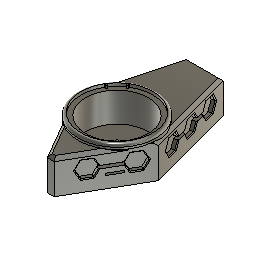
wedge_15deg_18mm_cirque (Autodesk Fusion 360 design; units mm, degrees)
Autodesk Fusion 360 part; units mm, degrees
sketch "wedge-base" plane through (0, 0, 0) normal (0, 0, 1) x (1, 0, 0)
  line L0 (-31.305, -84.6876) -> (-19.8752, -42.031)
  line L1 (-139.1957, -104.8346) -> (-25.4147, -135.3221)
  line L2 (-74.9975, -19.3163) -> (-95.8937, -18.9648)
  line L3 (-118.0318, -25.8497) -> (-139.1957, -104.8346)
  line L4 (-95.8937, -18.9648) -> (-118.0318, -25.8497)
  line L5 (-12.6022, -117.024) -> (-31.305, -84.6876)
  line L6 (-19.8752, -42.031) -> (-56.3483, -24.332)
  line L7 (-56.3483, -24.332) -> (-56.434, -24.2904)
  line L8 (-25.4147, -135.3221) -> (-12.6022, -117.024)
  line L9 (-56.434, -24.2904) -> (-74.9975, -19.3163)
  line L10 (-55.3814, -21.4666) -> (-74.5778, -16.323)
  line L11 (-24.1621, -138.7635) -> (-9.0476, -117.1778)
  line L12 (-120.5016, -23.4761) -> (-142.8699, -106.9559)
  line L13 (-16.336, -40.4139) -> (-55.3814, -21.4666)
  line L14 (-74.5778, -16.323) -> (-96.3248, -15.9571)
  line L15 (-9.0476, -117.1778) -> (-28.0852, -84.2624)
  line L16 (-28.0852, -84.2624) -> (-16.336, -40.4139)
  line L17 (-96.3248, -15.9571) -> (-120.5016, -23.4761)
  line L18 (-142.8699, -106.9559) -> (-24.1621, -138.7635)
  line L19 (-30.0171, -84.5175) -> (-18.4595, -41.3841)
  line L20 (-119.0197, -24.9003) -> (-140.6654, -105.6831)
  line L21 (-24.9136, -136.6987) -> (-11.1804, -117.0855)
  line L22 (-96.0662, -17.7617) -> (-119.0197, -24.9003)
  line L23 (-18.4595, -41.3841) -> (-56.013, -23.1609)
  line L24 (-140.6654, -105.6831) -> (-24.9136, -136.6987)
  line L25 (-56.013, -23.1609) -> (-74.8297, -18.119)
  line L26 (-11.1804, -117.0855) -> (-30.0171, -84.5175)
  line L27 (-74.8297, -18.119) -> (-96.0662, -17.7617)
  line L28 (-55.5625, -22.7126) -> (-55.8025, -22.5961)
  line L29 (-29.3731, -84.4325) -> (-17.7517, -41.0607)
  line L30 (-55.8025, -22.5961) -> (-74.7457, -17.5203)
  line L31 (-17.7517, -41.0607) -> (-55.5625, -22.7126)
  line L32 (-74.7457, -17.5203) -> (-96.1524, -17.1602)
  line L33 (-119.5136, -24.4255) -> (-141.4002, -106.1074)
  line L34 (-10.4694, -117.1163) -> (-29.3731, -84.4325)
  line L35 (-141.4002, -106.1074) -> (-24.6631, -137.387)
  line L36 (-24.6631, -137.387) -> (-10.4694, -117.1163)
  line L37 (-96.1524, -17.1602) -> (-119.5136, -24.4255)
  circle A0 centre (-97.5457, -40.1917) radius 2.2
  circle A1 centre (-107.3808, -76.8969) radius 2.2
  circle A2 centre (-47.3176, -53.6503) radius 2.2
  circle A3 centre (-43.0743, -100.1574) radius 2.2
  line L38 (-104.5834, -110.8892) -> (-99.9246, -93.5026)
  line L39 (-136.4589, -102.3482) -> (-104.5834, -110.8892)
  line L40 (-99.9246, -93.5026) -> (-131.8002, -84.9615)
  line L41 (-131.8002, -84.9615) -> (-136.4589, -102.3482)
  line L42 (-100.5004, -109.2708) -> (-102.0145, -114.9215)
  line L43 (-93.5143, -117.1991) -> (-92.0002, -111.5484)
  line L44 (-92.0002, -111.5484) -> (-100.5004, -109.2708)
  line L45 (-82.5358, -118.7276) -> (-81.63, -115.3469)
  line L46 (-90.3233, -113.0175) -> (-91.2292, -116.3983)
  line L47 (-81.63, -115.3469) -> (-90.3233, -113.0175)
  line L48 (-91.2292, -116.3983) -> (-82.5358, -118.7276)
  line L49 (-21.0709, -104.8602) -> (-26.5709, -95.3339)
  line L50 (-28.9517, -109.4102) -> (-21.0709, -104.8602)
  line L51 (-26.5709, -95.3339) -> (-34.4517, -99.8839)
  line L52 (-34.4517, -99.8839) -> (-28.9517, -109.4102)
  line L53 (-107.7035, -88.1467) -> (-99.3965, -90.3726)
  line L54 (-99.3965, -90.3726) -> (-97.093, -81.7758)
  line L55 (-97.093, -81.7758) -> (-105.4, -79.55)
  line L56 (-105.4, -79.55) -> (-107.7035, -88.1467)
  line L57 (-7.336, -20.2677) -> (-7.336, -143.1078) construction
  line L58 (3.7874, -41.3841) -> (41.3409, -23.1609)
  line L59 (126.7282, -106.1074) -> (9.991, -137.387)
  line L60 (-7.336, -20.2677) -> (-7.336, -143.1078) construction
  line L61 (10.2415, -136.6987) -> (-3.4917, -117.0855)
  line L62 (41.1304, -22.5961) -> (60.0736, -17.5203)
  line L63 (11.8988, -95.3339) -> (19.7796, -99.8839)
  line L64 (105.8295, -23.4761) -> (128.1978, -106.9559)
  line L65 (19.7796, -99.8839) -> (14.2796, -109.4102)
  line L66 (41.3409, -23.1609) -> (60.1576, -18.119)
  line L67 (15.345, -84.5175) -> (3.7874, -41.3841)
  line L68 (40.7094, -21.4666) -> (59.9057, -16.323)
  line L69 (78.8422, -117.1991) -> (77.3281, -111.5484)
  line L70 (-3.4917, -117.0855) -> (15.345, -84.5175)
  line L71 (76.5571, -116.3983) -> (67.8638, -118.7276)
  line L72 (-4.2026, -117.1163) -> (14.7011, -84.4325)
  line L73 (16.6329, -84.6876) -> (5.2031, -42.031)
  line L74 (85.2525, -93.5026) -> (117.1281, -84.9615)
  line L75 (81.3941, -17.7617) -> (104.3476, -24.9003)
  line L76 (75.6512, -113.0175) -> (76.5571, -116.3983)
  line L77 (66.9579, -115.3469) -> (75.6512, -113.0175)
  circle A4 centre (32.6455, -53.6503) radius 2.2
  line L78 (89.9113, -110.8892) -> (85.2525, -93.5026)
  line L79 (14.7011, -84.4325) -> (3.0796, -41.0607)
  line L80 (67.8638, -118.7276) -> (66.9579, -115.3469)
  line L81 (128.1978, -106.9559) -> (9.49, -138.7635)
  line L82 (81.4803, -17.1602) -> (104.8416, -24.4255)
  line L83 (13.4132, -84.2624) -> (1.664, -40.4139)
  circle A5 centre (92.7087, -76.8969) radius 2.2
  line L84 (10.7426, -135.3221) -> (-2.0699, -117.024)
  line L85 (93.0314, -88.1467) -> (84.7244, -90.3726)
  line L86 (104.3476, -24.9003) -> (125.9933, -105.6831)
  line L87 (1.664, -40.4139) -> (40.7094, -21.4666)
  line L88 (90.7279, -79.55) -> (93.0314, -88.1467)
  line L89 (81.2217, -18.9648) -> (103.3597, -25.8497)
  line L90 (3.0796, -41.0607) -> (40.8904, -22.7126)
  line L91 (125.9933, -105.6831) -> (10.2415, -136.6987)
  line L92 (-2.0699, -117.024) -> (16.6329, -84.6876)
  line L93 (84.7244, -90.3726) -> (82.421, -81.7758)
  line L94 (81.6527, -15.9571) -> (105.8295, -23.4761)
  line L95 (9.991, -137.387) -> (-4.2026, -117.1163)
  line L96 (121.7868, -102.3482) -> (89.9113, -110.8892)
  line L97 (60.0736, -17.5203) -> (81.4803, -17.1602)
  line L98 (59.9057, -16.323) -> (81.6527, -15.9571)
  line L99 (6.3988, -104.8602) -> (11.8988, -95.3339)
  line L100 (82.421, -81.7758) -> (90.7279, -79.55)
  circle A6 centre (28.4022, -100.1574) radius 2.2
  line L101 (60.1576, -18.119) -> (81.3941, -17.7617)
  line L102 (41.6762, -24.332) -> (41.7619, -24.2904)
  line L103 (9.49, -138.7635) -> (-5.6245, -117.1778)
  line L104 (41.7619, -24.2904) -> (60.3255, -19.3163)
  circle A7 centre (82.8736, -40.1917) radius 2.2
  line L105 (40.8904, -22.7126) -> (41.1304, -22.5961)
  line L106 (-5.6245, -117.1778) -> (13.4132, -84.2624)
  line L107 (124.5236, -104.8346) -> (10.7426, -135.3221)
  line L108 (117.1281, -84.9615) -> (121.7868, -102.3482)
  line L109 (14.2796, -109.4102) -> (6.3988, -104.8602)
  line L110 (104.8416, -24.4255) -> (126.7282, -106.1074)
  line L111 (103.3597, -25.8497) -> (124.5236, -104.8346)
  line L112 (5.2031, -42.031) -> (41.6762, -24.332)
  line L113 (77.3281, -111.5484) -> (85.8283, -109.2708)
  line L114 (85.8283, -109.2708) -> (87.3424, -114.9215)
  line L115 (60.3255, -19.3163) -> (81.2217, -18.9648)
  line L116 (-28.0852, -84.2624) -> (13.4132, -84.2624) construction
  line L117 (-16.336, -40.4139) -> (1.664, -40.4139)
  line L118 (-9.0476, -117.1778) -> (-5.6245, -117.1778)
  point P0 (-7.336, -84.2624)
  dimension "d1" = 9
  dimension "d2" = 9
  constraint vertical L57
  constraint horizontal L116
  constraint midpoint L116 P0
  constraint coincident L13.start L16.end
  constraint perpendicular L57 L117
  constraint parallel L117 L118
  measures "d1" distance of L13.start L57
  measures "d2" distance of L83.end L60
extrude "Extrude1" add sketch "wedge-base" along normal blind 16.6 contours L15 L16 L83 L106 L117 L118
sketch "cirque" plane through (0, 0, 0) normal (0, 0, 1) x (1, 0, 0)
  arc A0 (-17.2299, -69.4279) -> (-22.1706, -74.3686) centre (-7.336, -84.2624) ccw
  arc A1 (4.4021, -96.566) -> (4.9675, -96.0005) centre (4.6848, -96.2833) cw
  arc A2 (-21.4728, -74.8131) -> (-21.8745, -75.4436) centre (-21.6737, -75.1283) cw
  arc A3 (-16.1549, -69.7239) -> (-16.7854, -70.1256) centre (-16.4701, -69.9248) cw
  line L0 (4.9675, -96.0005) -> (5.5521, -96.5851)
  arc A4 (-22.5723, -74.9991) -> (4.9867, -97.1506) centre (-7.336, -84.2624) ccw
  line L1 (-22.1706, -74.3686) -> (-21.4728, -74.8131)
  line L2 (-16.7854, -70.1256) -> (-17.2299, -69.4279)
  line L3 (4.9867, -97.1506) -> (4.4021, -96.566)
  line L4 (-21.8745, -75.4436) -> (-22.5723, -74.9991)
  arc A5 (5.5521, -96.5851) -> (-16.5994, -69.0262) centre (-7.336, -84.2624) ccw
  line L5 (-16.5994, -69.0262) -> (-16.1549, -69.7239)
  circle A6 centre (-7.336, -84.2624) radius 15.5
  line L6 (-7.336, -66.2625) -> (-7.336, -66.5624)
  circle A7 centre (-7.336, -84.2624) radius 19.3
  point P0 (-7.336, -84.2624)
  dimension "d3" = 3.8
extrude "Extrude2" cut sketch "cirque" along normal up to surface (13.6 mm away) from surface at 3 contours A6
extrude "Extrude3" add sketch "cirque" along normal blind 1 from surface at 16.6 contours A0 A1 A2 A3 L0 A4 L1 L2 L3 L4 A5 L5
extrude "Extrude5" add sketch "cirque" along normal blind 2.5 from surface at 16.6 contours A7
sketch "Sketch6" plane through (46.5701, -26.9353, 0) normal (0.865639, -0.500669, 0) x (0.500669, 0.865639, 0)
  line L0 (-104.2497, 0) -> (-66.2253, 0)
  line L1 (-66.2253, 0) -> (-66.2253, 16.6)
  line L2 (-66.2253, 16.6) -> (-69.5511, 16.6)
  line L3 (-69.5511, 16.6) -> (-83.6764, 16.6)
  line L4 (-83.6764, 16.6) -> (-104.2497, 16.6)
  line L5 (-104.2497, 16.6) -> (-104.2497, 0)
  line L6 (-85.5673, 5.7) -> (-85.5673, 6.7)
  line L7 (-85.5673, 6.7) -> (-78.5673, 6.7)
  line L8 (-78.5673, 5.7) -> (-85.5673, 5.7)
  line L9 (-78.5673, 6.7) -> (-78.5673, 5.7)
  line L10 (-104.2497, 16.6) -> (-104.2497, 2)
  line L11 (-104.2497, 2) -> (-66.2253, 2)
  line L12 (-66.2253, 16.6) -> (-104.2497, 16.6)
  line L13 (-66.2253, 2) -> (-66.2253, 16.6)
  line L14 (-89.961, 5.7214) -> (-87.6598, 9.6927)
  line L15 (-94.5383, 13.6786) -> (-96.8396, 9.7073)
  line L16 (-87.6598, 9.6927) -> (-89.9484, 13.6713)
  line L17 (-96.8396, 9.7073) -> (-94.551, 5.7287)
  line L18 (-94.551, 5.7287) -> (-89.961, 5.7214)
  line L19 (-89.9484, 13.6713) -> (-94.5383, 13.6786)
  line L20 (-71.9366, 13.6786) -> (-76.5266, 13.6713)
  line L21 (-69.6354, 9.7073) -> (-71.9366, 13.6786)
  line L22 (-71.924, 5.7287) -> (-69.6354, 9.7073)
  line L23 (-78.8152, 9.6927) -> (-76.5139, 5.7214)
  line L24 (-76.5266, 13.6713) -> (-78.8152, 9.6927)
  line L25 (-76.5139, 5.7214) -> (-71.924, 5.7287)
  arc A0 (-92.2497, 10.45) -> (-92.2497, 8.95) centre (-92.2497, 9.7) ccw
  line L26 (-92.2497, 8.95) -> (-74.2253, 8.95)
  line L27 (-74.2253, 10.45) -> (-92.2497, 10.45)
  arc A1 (-74.2253, 8.95) -> (-74.2253, 10.45) centre (-74.2253, 9.7) ccw
  point P0 (-92.2497, 9.7)
  point P1 (-74.2253, 9.7)
  point P2 (-92.2497, 9.7)
  point P3 (-74.2253, 9.7)
sketch "Sketch8" plane through (-57.5643, -33.2941, 0) normal (-0.865639, -0.500669, 0) x (0.500669, -0.865639, 0)
  line L0 (58.8794, 0) -> (96.9038, 0)
  line L1 (96.9038, 0) -> (96.9038, 16.6)
  line L2 (96.9038, 16.6) -> (76.3306, 16.6)
  line L3 (76.3306, 16.6) -> (62.2052, 16.6)
  line L4 (62.2052, 16.6) -> (58.8794, 16.6)
  line L5 (58.8794, 16.6) -> (58.8794, 0)
  line L6 (58.8794, 2) -> (58.8794, 16.6)
  line L7 (58.8794, 16.6) -> (96.9038, 16.6)
  line L8 (96.9038, 2) -> (58.8794, 2)
  line L9 (58.8794, 2) -> (58.8794, 16.6)
  line L10 (66.8794, 10.45) -> (84.9038, 10.45)
  line L11 (78.2215, 6.7) -> (71.2215, 6.7)
  line L12 (84.9038, 8.95) -> (66.8794, 8.95)
  line L13 (82.6152, 5.7214) -> (80.3139, 9.6927)
  line L14 (89.4938, 9.7073) -> (87.2051, 5.7287)
  arc A0 (66.8794, 8.95) -> (66.8794, 10.45) centre (66.8794, 9.7) cw
  line L15 (71.2215, 6.7) -> (71.2215, 5.7)
  line L16 (78.2215, 5.7) -> (78.2215, 6.7)
  line L17 (71.2215, 5.7) -> (78.2215, 5.7)
  line L18 (69.1807, 13.6713) -> (71.4694, 9.6927)
  line L19 (64.5781, 5.7287) -> (62.2895, 9.7073)
  line L20 (87.2051, 5.7287) -> (82.6152, 5.7214)
  line L21 (71.4694, 9.6927) -> (69.1681, 5.7214)
  line L22 (87.1925, 13.6786) -> (89.4938, 9.7073)
  line L23 (62.2895, 9.7073) -> (64.5908, 13.6786)
  line L24 (82.6025, 13.6713) -> (87.1925, 13.6786)
  line L25 (64.5908, 13.6786) -> (69.1807, 13.6713)
  line L26 (96.9038, 16.6) -> (96.9038, 2)
  line L27 (80.3139, 9.6927) -> (82.6025, 13.6713)
  arc A1 (84.9038, 10.45) -> (84.9038, 8.95) centre (84.9038, 9.7) cw
  line L28 (69.1681, 5.7214) -> (64.5781, 5.7287)
  point P0 (84.9038, 9.7)
  point P1 (66.8794, 9.7)
  point P2 (66.8794, 9.7)
  point P3 (84.9038, 9.7)
sketch "Sketch9" plane through (-8.551, -2.2912, 0) normal (0.965926, 0.258819, 0) x (-0.258819, 0.965926, 0)
  line L0 (-84.8628, 0) -> (-39.4675, 0)
  line L1 (-39.4675, 0) -> (-39.4675, 16.6)
  line L2 (-39.4675, 16.6) -> (-84.8628, 16.6)
  line L3 (-84.8628, 16.6) -> (-84.8628, 0)
  line L4 (-84.8628, 16.6) -> (-84.8628, 2)
  line L5 (-39.4675, 16.6) -> (-84.8628, 16.6)
  line L6 (-84.8628, 2) -> (-39.4675, 2)
  line L7 (-39.4675, 2) -> (-39.4675, 16.6)
  line L8 (-77.4793, 5.7361) -> (-72.8894, 5.714)
  line L9 (-72.851, 13.6639) -> (-77.4409, 13.686)
  line L10 (-72.8894, 5.714) -> (-70.5753, 9.6778)
  line L11 (-77.4409, 13.686) -> (-79.755, 9.7222)
  line L12 (-70.5753, 9.6778) -> (-72.851, 13.6639)
  line L13 (-79.755, 9.7222) -> (-77.4793, 5.7361)
  line L14 (-64.4409, 13.686) -> (-66.755, 9.7222)
  line L15 (-59.851, 13.6639) -> (-64.4409, 13.686)
  line L16 (-64.4793, 5.7361) -> (-59.8894, 5.714)
  line L17 (-66.755, 9.7222) -> (-64.4793, 5.7361)
  line L18 (-59.8894, 5.714) -> (-57.5753, 9.6778)
  line L19 (-57.5753, 9.6778) -> (-59.851, 13.6639)
  line L20 (-46.8894, 5.714) -> (-44.5753, 9.6778)
  line L21 (-46.851, 13.6639) -> (-51.4409, 13.686)
  line L22 (-44.5753, 9.6778) -> (-46.851, 13.6639)
  line L23 (-51.4793, 5.7361) -> (-46.8894, 5.714)
  line L24 (-51.4409, 13.686) -> (-53.755, 9.7222)
  line L25 (-53.755, 9.7222) -> (-51.4793, 5.7361)
  line L26 (-75.1651, 8.95) -> (-49.1651, 8.95)
  arc A0 (-49.1651, 8.95) -> (-49.1651, 10.45) centre (-49.1651, 9.7) ccw
  line L27 (-49.1651, 10.45) -> (-75.1651, 10.45)
  arc A1 (-75.1651, 10.45) -> (-75.1651, 8.95) centre (-75.1651, 9.7) ccw
  point P0 (-62.1651, 9.7)
  point P1 (-49.1651, 9.7)
  point P2 (-75.1651, 9.7)
  point P3 (-75.1651, 9.7)
  point P4 (-62.1651, 9.7)
  point P5 (-49.1651, 9.7)
sketch "Sketch10" plane through (-5.1383, 1.3768, 0) normal (-0.965926, 0.258819, 0) x (-0.258819, -0.965926, 0)
  line L0 (43.2649, 0) -> (88.6603, 0)
  line L1 (88.6603, 0) -> (88.6603, 16.6)
  line L2 (88.6603, 16.6) -> (43.2649, 16.6)
  line L3 (43.2649, 16.6) -> (43.2649, 0)
  line L4 (43.2649, 2) -> (88.6603, 2)
  line L5 (43.2649, 16.6) -> (43.2649, 2)
  line L6 (88.6603, 2) -> (88.6603, 16.6)
  line L7 (88.6603, 16.6) -> (43.2649, 16.6)
  line L8 (50.6484, 5.7361) -> (55.2383, 5.714)
  line L9 (48.3727, 9.7222) -> (50.6484, 5.7361)
  line L10 (50.6868, 13.686) -> (48.3727, 9.7222)
  line L11 (55.2767, 13.6639) -> (50.6868, 13.686)
  line L12 (55.2383, 5.714) -> (57.5524, 9.6778)
  line L13 (57.5524, 9.6778) -> (55.2767, 13.6639)
  line L14 (68.2383, 5.714) -> (70.5524, 9.6778)
  line L15 (63.6484, 5.7361) -> (68.2383, 5.714)
  line L16 (70.5524, 9.6778) -> (68.2767, 13.6639)
  line L17 (61.3727, 9.7222) -> (63.6484, 5.7361)
  line L18 (63.6868, 13.686) -> (61.3727, 9.7222)
  line L19 (68.2767, 13.6639) -> (63.6868, 13.686)
  line L20 (74.3727, 9.7222) -> (76.6484, 5.7361)
  line L21 (76.6484, 5.7361) -> (81.2383, 5.714)
  line L22 (83.5524, 9.6778) -> (81.2767, 13.6639)
  line L23 (76.6868, 13.686) -> (74.3727, 9.7222)
  line L24 (81.2767, 13.6639) -> (76.6868, 13.686)
  line L25 (81.2383, 5.714) -> (83.5524, 9.6778)
  line L26 (78.9626, 10.45) -> (52.9626, 10.45)
  line L27 (52.9626, 8.95) -> (78.9626, 8.95)
  arc A0 (78.9626, 8.95) -> (78.9626, 10.45) centre (78.9626, 9.7) ccw
  arc A1 (52.9626, 10.45) -> (52.9626, 8.95) centre (52.9626, 9.7) ccw
  point P0 (65.9626, 9.7)
  point P1 (78.9626, 9.7)
  point P2 (52.9626, 9.7)
  point P3 (52.9626, 9.7)
  point P4 (65.9626, 9.7)
  point P5 (78.9626, 9.7)
extrude "Extrude8" cut sketch "Sketch6" along normal up to surface contours L6 L7 L8 L9 end surface at (8.1447, -85.0351, 12.7333)
extrude "Extrude9" cut sketch "Sketch8" along normal up to surface contours L11 L15 L16 L17 end surface at (-2.8574, -99.1013, 9.1)
extrude "Extrude10" cut sketch "Sketch8" against normal blind 2 contours L10 L12 A0 L18 L19 L21 L23 L25 L28 | L10 L12 A0 L18 L21 | L10 L12 L13 L18 L21 L27 | L10 L12 L13 L14 L20 L22 L24 L27 A1 | L10 L12 L13 L27 A1
extrude "Extrude11" cut sketch "Sketch10" against normal blind 2 contours L8 L9 L10 L11 L12 L13 L26 L27 A1 | L12 L13 L26 L27 A1 | L12 L13 L17 L18 L26 L27 | L14 L15 L17 L27 | L14 L16 L17 L18 L26 L27 | L14 L16 L20 L23 L26 L27 | L16 L18 L19 L26 | L20 L21 L22 L23 L24 L25 L26 L27 A0 | L20 L23 L26 L27 A0
extrude "Extrude12" cut sketch "Sketch9" against normal blind 2 contours L8 L9 L10 L11 L12 L13 L26 L27 A1 | L10 L12 L26 L27 A1 | L10 L12 L14 L17 L26 L27 | L16 L17 L18 L26 | L14 L17 L18 L19 L26 L27 | L18 L19 L24 L25 L26 L27 | L14 L15 L19 L27 | L20 L21 L22 L23 L24 L25 L26 A0 L27 | L24 L25 L26 A0 L27
extrude "Extrude13" cut sketch "Sketch6" against normal blind 2 contours L14 L15 L16 L17 L18 L19 A0 L26 L27 | L14 L16 A0 L26 L27 | L14 L16 L23 L24 L26 L27 | L20 L21 L22 L23 L24 L25 L26 L27 A1 | L23 L24 L26 L27 A1
chamfer "Chamfer7" distance 0.4 angle 45 60 edges at (0.3867, -106.7847, 13.675) (-1.3384, -109.7674, 11.693) (-1.3416, -109.7728, 7.718) (0.3804, -106.7956, 5.725) (1.9977, -103.9993, 7.3357) (1.9996, -103.9961, 12.0607) (7.7917, -93.9817, 12.0607) (9.4046, -91.193, 13.675) (11.1297, -88.2104, 11.693) (11.1329, -88.2049, 7.718) (9.411, -91.1821, 5.725) (7.7936, -93.9785, 7.3357) (11.7917, -78.211, 11.7041) (11.7966, -78.2296, 7.7291) (10.9082, -74.9137, 5.725) (10.0697, -71.7846, 7.332) (10.0668, -71.7737, 12.0569) (10.8982, -74.8767, 13.675) (8.372, -65.4488, 12.068) (7.5336, -62.3196, 13.675) (6.7022, -59.2167, 12.0569) (6.7051, -59.2275, 7.332) (7.5435, -62.3567, 5.725) (8.375, -65.4596, 7.3431) (5.0074, -52.8917, 12.068) (4.1689, -49.7626, 13.675) (3.2805, -46.4467, 11.6709) (3.2854, -46.4653, 7.6959) (4.1789, -49.7996, 5.725) (5.0103, -52.9026, 7.3431) (-18.851, -49.7996, 13.675) (-17.9575, -46.4653, 11.7041) (-17.9525, -46.4467, 7.7291) (-18.841, -49.7626, 5.725) (-19.6795, -52.8917, 7.332) (-19.6824, -52.9026, 12.0569) (-21.3771, -59.2275, 12.068) (-21.3742, -59.2167, 7.3431) (-22.2057, -62.3196, 5.725) (-23.0441, -65.4488, 7.332) (-23.047, -65.4596, 12.0569) (-22.2156, -62.3567, 13.675) (-24.7418, -71.7846, 12.068) (-25.5802, -74.9137, 13.675) (-26.4687, -78.2296, 11.6709) (-26.4638, -78.211, 7.6959) (-25.5703, -74.8767, 5.725) (-24.7389, -71.7737, 7.3431) (-24.0767, -91.193, 13.675) (-25.8018, -88.2104, 11.693) (-25.805, -88.2049, 7.718) (-24.083, -91.1821, 5.725) (-22.4657, -93.9785, 7.3357) (-22.4638, -93.9817, 12.0607) (-16.6717, -103.9961, 12.0607) (-16.6698, -103.9993, 7.3357) (-15.0525, -106.7956, 5.725) (-13.3305, -109.7728, 7.718) (-13.3337, -109.7674, 11.693) (-15.0588, -106.7847, 13.675)
fillet "Fillet1" radius 1.5 1 edges at (-25.33, -91.2416, 19.1)
chamfer "Chamfer1" distance 1.5 angle 45 6 edges at (-14.1978, -108.2733, 16.6) (-7.336, -117.1778, 16.6) (-0.4743, -108.2733, 16.6) (-22.2106, -62.3381, 16.6) (-7.336, -40.4139, 16.6) (7.5386, -62.3381, 16.6)
chamfer "Chamfer2" distance 3.3 angle 45 2 edges at (-19.348, -99.3688, 15.85) (4.6759, -99.3688, 15.85)
chamfer "Chamfer3" distance 3 angle 45 2 edges at (-21.0002, -96.5122, 15.85) (6.3281, -96.5122, 15.85)
equation "d3 = 2.3 mm + 1.5 mm"
